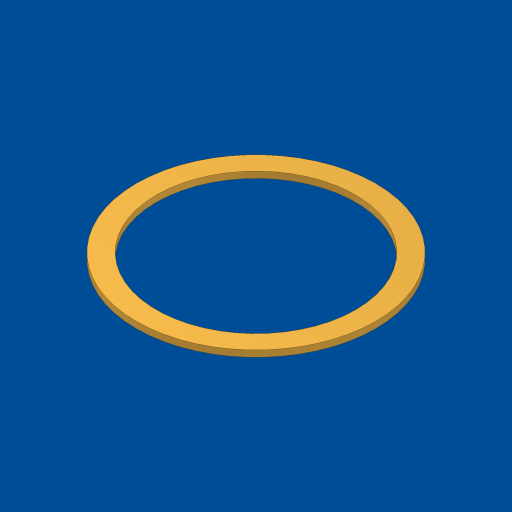
# Autodesk Inventor part: rp-sma_washer
Saved by Autodesk Inventor 2023.2 (Build 272271000, 271)
## iProperties
Created: 2023-01-27
Part Number: rp-sma_washer
Material: Brass, Soft Yellow
Document SubType Name: Modeling
Designer: agmlego
Mass: 0.0461035 g
Surface Area: 0.572602 cm^2
Volume: 0.00544315 cm^3
Density: 8.47 g/cm^3
Appearance: Brass - Satin
Author: agmlego
Autodesk Inventor part; units mm, degrees
ref_plane "YZ Plane" through (0, 0, 0) normal (1, 0, 0) x (0, 1, 0)
ref_plane "XZ Plane" through (0, 0, 0) normal (0, 1, 0) x (-1, 0, 0)
ref_plane "XY Plane" through (0, 0, 0) normal (0, 0, 1) x (1, 0, 0)
sketch "Sketch1" plane through (0, 0, 0) normal (0, 1, 0) x (-1, 0, 0)
  circle A0 centre (0, 0) radius 4.7625
  circle A1 centre (0, 0) radius 3.9688
  dimension "d0" = 9.525
  dimension "d1" = 7.9375
  constraints: 2 centre point, 2 coincident
  measures "d0" diameter of A0
  measures "d1" diameter of A1
extrude "Extrusion1" add sketch "Sketch1" along normal blind 0.25
body "Solid1"
